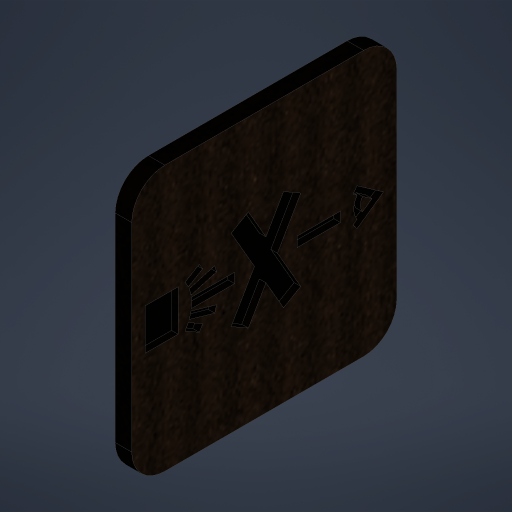
# Autodesk Inventor part: LightGateCard_V1
Saved by Autodesk Inventor 2024.1 (Build 281209000, 209)
## iProperties
Created: 2023-05-21
Part Number: LightGateCard_V1
Material: MDF Medium Density Fiberboard
Document SubType Name: Modeling
Designer: jaege
Density: 0.8 g/cm^3
Appearance: Cardboard - Corrugated
Mass: 4.78727 g
Surface Area: 45.5722 cm^2
Volume: 5.98408 cm^3
Author: jaege
## iProperties of the stored document LightGateCard_3DPrint.ipt
Created: 2023-08-10
Part Number: LightGateCard_3DPrint
Material: Generic
Document SubType Name: Modeling
Designer: jaege
Density: 1 g/cm^3
Appearance: Default
Author: jaege
Autodesk Inventor part; units mm, degrees
ref_plane "YZ Plane" through (0, 0, 0) normal (1, 0, 0) x (0, 1, 0)
ref_plane "XZ Plane" through (0, 0, 0) normal (0, 1, 0) x (-1, 0, 0)
ref_plane "XY Plane" through (0, 0, 0) normal (0, 0, 1) x (1, 0, 0)
sketch "Sketch1" plane through (0, 0, 0) normal (1, 0, 0) x (0, 1, 0)
  line L0 (-20, -20) -> (20, -20)
  line L1 (20, -20) -> (20, 20)
  line L2 (20, 20) -> (-20, 20)
  line L3 (-20, 20) -> (-20, -20)
  line L4 (-20, -20) -> (20, 20) construction
  line L5 (20, -20) -> (-20, 20) construction
  point P0 (0, 0)
  dimension "d1" = 40
  dimension "d2" = 40
  constraints: 12 end point, 2 midpoint, 2 parallel, 1 horizontal, 1 perpendicular
  measures "d1" distance of L0.start L0.end
  measures "d2" distance of L0.end L1.end
extrude "Outline" add sketch "Sketch1" along normal blind 2.5
sketch "Sketch2" plane through (2.5, 0, 0) normal (1, 0, 0) x (0, 0, -1)
  line L0 (20, 20) -> (-20, 20) projected
  line L1 (20, -20) -> (20, 20) projected
  line L2 (-18, 3.1) -> (-13, 3.1)
  line L3 (-13, 3.1) -> (-13, -3.1)
  line L4 (-13, -3.1) -> (-18, -3.1)
  line L5 (-18, -3.1) -> (-18, 3.1)
  line L6 (-11, 0.75) -> (-4.4788, 0.75)
  line L7 (-4.4788, 0.75) -> (-4.4788, -0.75)
  line L8 (-4.4788, -0.75) -> (-11, -0.75)
  line L9 (-11, -0.75) -> (-11, 0.75)
  line L10 (13.9738, 2.8192) -> (18, 0)
  line L11 (18, 0) -> (13.9738, -2.8192)
  line L12 (13.9738, 2.8192) -> (13.4003, 2)
  line L13 (13.4003, 2) -> (16.2566, 0)
  line L14 (16.2566, 0) -> (13.4003, -2)
  line L15 (13.4003, -2) -> (13.9738, -2.8192)
  line L16 (-18, 0) -> (16.2566, 0) construction
  arc A0 (14.0039, 1.5773) -> (14.0039, -1.5773) centre (16.2566, 0) ccw
  arc A1 (14.823, 1.0038) -> (14.823, -1.0038) centre (16.2566, 0) ccw
  line L17 (4.9853, 0.75) -> (11.5066, 0.75)
  line L18 (11.5066, 0.75) -> (11.5066, -0.75)
  line L19 (11.5066, -0.75) -> (4.9853, -0.75)
  line L20 (4.9853, -0.75) -> (4.9853, 0.75)
  line L21 (-11.3236, 2.0044) -> (-11.048, 1.0432)
  line L22 (-11.048, 1.0432) -> (-7.203, 2.1457)
  line L23 (-7.203, 2.1457) -> (-7.4786, 3.107)
  line L24 (-7.4786, 3.107) -> (-11.3236, 2.0044)
  line L25 (-11.048, -1.0432) -> (-7.203, -2.1457)
  line L26 (-7.203, -2.1457) -> (-7.4786, -3.107)
  line L27 (-7.4786, -3.107) -> (-11.3236, -2.0044)
  line L28 (-11.3236, -2.0044) -> (-11.048, -1.0432)
  circle A2 centre (-16.5, 0) radius 5.5509 construction
  line L29 (-11.9623, 3.1972) -> (-11.4623, 2.3312)
  line L30 (-11.4623, 2.3312) -> (-9.2973, 3.5812)
  line L31 (-9.2973, 3.5812) -> (-9.7973, 4.4472)
  line L32 (-9.7973, 4.4472) -> (-11.9623, 3.1972)
  line L33 (-11.4623, -2.3312) -> (-11.9623, -3.1972)
  line L34 (-11.9623, -3.1972) -> (-9.7973, -4.4472)
  line L35 (-9.7973, -4.4472) -> (-9.2973, -3.5812)
  line L36 (-9.2973, -3.5812) -> (-11.4623, -2.3312)
  line L37 (-4.9984, 6.0961) -> (-2.4003, 7.5961)
  line L38 (-2.4003, 7.5961) -> (5.5049, -6.0961)
  line L39 (5.5049, -6.0961) -> (2.9068, -7.5961)
  line L40 (2.9068, -7.5961) -> (-4.9984, 6.0961)
  line L41 (-4.9984, -6.0961) -> (2.9068, 7.5961)
  line L42 (2.9068, 7.5961) -> (5.5049, 6.0961)
  line L43 (5.5049, 6.0961) -> (-2.4003, -7.5961)
  line L44 (-2.4003, -7.5961) -> (-4.9984, -6.0961)
  line L45 (-4.9984, 7.5961) -> (5.5049, 7.5961) construction
  line L46 (5.5049, 7.5961) -> (5.5049, -7.5961) construction
  line L47 (5.5049, -7.5961) -> (-4.9984, -7.5961) construction
  line L48 (-4.9984, -7.5961) -> (-4.9984, 7.5961) construction
  line L49 (-20, -20) -> (20, -20) projected
  line L50 (-20, 20) -> (-20, -20) projected
  line L51 (-4.9984, 6.0961) -> (-11, 6.0961) construction
  line L52 (5.5049, 6.0961) -> (11.5066, 6.0961) construction
  point P0 (0, 0)
  point P1 (-13, 0)
  point P2 (-11, 0)
  point P3 (13.5066, 0)
  point P4 (-1.0458, 0.75)
  point P5 (1.5523, 0.75)
  point P6 (0.2533, -7.5961)
  point P7 (11.5066, 0)
  point P8 (5.5049, 0)
  point P9 (4.9853, 0)
  point P10 (-1.4788, 0)
  point P11 (0.2533, -3)
  point P12 (1.9853, 0)
  point P13 (0.2533, 3)
  point P14 (20, 0)
  dimension "d12" = 35
  dimension "d13" = 35
  dimension "d14" = 4
  dimension "d15" = 1
  dimension "d16" = 1
  dimension "d17" = 2.75
  dimension "d18" = 1.5
  dimension "d19" = 2
  dimension "d21" = 5
  dimension "d22" = 2
  dimension "d23" = 1
  dimension "d24" = 1
  dimension "d25" = 3.5
  dimension "d26" = 16
  dimension "d27" = 16
  dimension "d28" = 4
  dimension "d29" = 2.5
  dimension "d30" = 1
  dimension "d31" = 14
  dimension "d32" = 14
  dimension "d33" = 1
  dimension "d34" = 2.5
  dimension "d35" = 6.2
  dimension "d36" = 60
  dimension "d37" = 60
  dimension "d38" = 3
  dimension "d40" = 2
  dimension "d41" = 2
  dimension "d42" = 3
  dimension "d45" = 15.1922
  constraints: 98 end point, 22 parallel, 12 perpendicular, 10 midpoint, 7 horizontal, 7 horizontal alignment, 7 point on line, 6 vertical alignment, 5 equal length, 5 point on circle, 2 centre point, 2 collinear, 1 concentric, 11 other
  measures "d12" angle of L10 L16
  measures "d13" angle of L11 L16
  measures "d14" distance of L14.end L13.start
  measures "d15" radial gap between concentric circles of A1 A0
  measures "d16" distance between parallel lines of L10 L13
  measures "d17" radius of A0
  measures "d18" distance of L8.end L6.start
  measures "d19" distance from line of point (13.507, 0) L18
  measures "d21" distance between parallel lines of L5 L3
  measures "d22" distance between parallel lines of L3 L9
  measures "d23" distance of L23.start L23.end
  measures "d24" distance of L26.start L26.end
  measures "d25" distance from line of L3 point (-16.5, 0)
  measures "d26" angle of L25 L8
  measures "d27" angle of L22 L6
  measures "d28" distance of L23.end L24.end
  measures "d29" distance of L31.start L29.end
  measures "d30" distance of L31.start L31.end
  measures "d31" angle of L24 L30
  measures "d32" angle of L27 L36
  measures "d33" distance of L35.start L36.start
  measures "d34" distance of L36.start L33.start
  measures "d35" distance of L4.end L2.start
  measures "d36" angle of L38 L41
  measures "d37" angle of L6 L41
  measures "d38" distance of L37.start L37.end
  measures "d40" distance between parallel lines of L50 L5
  measures "d41" distance from line of L1 L10.end
  measures "d42" distance from line of point (-1.479, 0) L7
  measures "d45" distance of L45.end L46.end
extrude "Extrusion2" cut sketch "Sketch2" against normal blind 1 contours L2 L3 L4 L5 | L6 L7 L8 L9 | L10 L11 L15 L14 L13 L12 | L13 A1 L14 A0 | L17 L18 L19 L20 | L24 L23 L22 L21 | L25 L26 L27 L28 | L32 L31 L30 L29 | L36 L35 L34 L33 | L37 L38 L41 L40 | L41 L38 L43 L40 | L40 L43 L44 L41 | L41 L42 L43 L38 | L43 L38 L39 L40
sketch "Sketch4" plane through (1.5, 0, 0) normal (1, 0, 0) x (0, 0, -1)
  line L0 (-11.3236, 2.0044) -> (-11.048, 1.0432) projected
  line L1 (-11.048, 1.0432) -> (-7.203, 2.1457) projected
  line L2 (-7.203, 2.1457) -> (-7.4786, 3.107) projected
  line L3 (-7.4786, 3.107) -> (-11.3236, 2.0044) projected
  line L4 (0.2533, -3) -> (2.9068, -7.5961) projected
  line L5 (2.9068, -7.5961) -> (5.5049, -6.0961) projected
  line L6 (5.5049, -6.0961) -> (1.9853, 0) projected
  line L7 (1.9853, 0) -> (5.5049, 6.0961) projected
  line L8 (5.5049, 6.0961) -> (2.9068, 7.5961) projected
  line L9 (2.9068, 7.5961) -> (0.2533, 3) projected
  line L10 (0.2533, 3) -> (-2.4003, 7.5961) projected
  line L11 (-2.4003, 7.5961) -> (-4.9984, 6.0961) projected
  line L12 (-4.9984, 6.0961) -> (-1.4788, 0) projected
  line L13 (-1.4788, 0) -> (-4.9984, -6.0961) projected
  line L14 (-4.9984, -6.0961) -> (-2.4003, -7.5961) projected
  line L15 (-2.4003, -7.5961) -> (0.2533, -3) projected
  line L16 (11.5066, 0.75) -> (4.9853, 0.75) projected
  line L17 (4.9853, 0.75) -> (4.9853, -0.75) projected
  line L18 (4.9853, -0.75) -> (11.5066, -0.75) projected
  line L19 (11.5066, -0.75) -> (11.5066, 0.75) projected
  line L20 (-9.2973, 3.5812) -> (-9.7973, 4.4472) projected
  line L21 (-9.7973, 4.4472) -> (-11.9623, 3.1972) projected
  line L22 (-11.9623, 3.1972) -> (-11.4623, 2.3312) projected
  line L23 (-11.4623, 2.3312) -> (-9.2973, 3.5812) projected
  line L24 (-4.4788, -0.75) -> (-4.4788, 0.75) projected
  line L25 (-4.4788, 0.75) -> (-11, 0.75) projected
  line L26 (-11, 0.75) -> (-11, -0.75) projected
  line L27 (-11, -0.75) -> (-4.4788, -0.75) projected
  line L28 (-9.7973, -4.4472) -> (-9.2973, -3.5812) projected
  line L29 (-9.2973, -3.5812) -> (-11.4623, -2.3312) projected
  line L30 (-11.4623, -2.3312) -> (-11.9623, -3.1972) projected
  line L31 (-11.9623, -3.1972) -> (-9.7973, -4.4472) projected
  line L32 (14.823, 1.0038) -> (16.2566, 0) projected
  line L33 (16.2566, 0) -> (14.823, -1.0038) projected
  arc A0 (14.823, 1.0038) -> (14.823, -1.0038) centre (16.2566, 0) ccw projected
  line L34 (13.9738, -2.8192) -> (18, 0) projected
  line L35 (18, 0) -> (13.9738, 2.8192) projected
  line L36 (13.9738, 2.8192) -> (13.4003, 2) projected
  line L37 (13.4003, 2) -> (14.0039, 1.5773) projected
  arc A1 (14.0039, 1.5773) -> (14.0039, -1.5773) centre (16.2566, 0) ccw projected
  line L38 (14.0039, -1.5773) -> (13.4003, -2) projected
  line L39 (13.4003, -2) -> (13.9738, -2.8192) projected
  line L40 (-11.3236, -2.0044) -> (-7.4786, -3.107) projected
  line L41 (-7.4786, -3.107) -> (-7.203, -2.1457) projected
  line L42 (-7.203, -2.1457) -> (-11.048, -1.0432) projected
  line L43 (-11.048, -1.0432) -> (-11.3236, -2.0044) projected
  line L44 (-13, -3.1) -> (-13, 3.1) projected
  line L45 (-13, 3.1) -> (-18, 3.1) projected
  line L46 (-18, 3.1) -> (-18, -3.1) projected
  line L47 (-18, -3.1) -> (-13, -3.1) projected
  line L48 (20, 20) -> (20, -20) projected
  line L49 (20, -20) -> (-20, -20) projected
  line L50 (-20, -20) -> (-20, 20) projected
  line L51 (-20, 20) -> (20, 20) projected
  point P0 (0, 0)
fillet "Fillet1" radius 5 4 edges at (1.25, 20, -20) (1.25, -20, -20) (1.25, 20, 20) (1.25, -20, 20)
sketch "Sketch5" plane through (2.5, 0, 0) normal (1, 0, 0) x (0, 0, -1)
  arc A0 (-20, -15) -> (-15, -20) centre (-15, -15) ccw projected
  line L0 (-20, -15) -> (-20, 15) projected
  arc A1 (-15, 20) -> (-20, 15) centre (-15, 15) ccw projected
  line L1 (-15, 20) -> (15, 20) projected
  arc A2 (20, 15) -> (15, 20) centre (15, 15) ccw projected
  line L2 (20, 15) -> (20, -15) projected
  arc A3 (15, -20) -> (20, -15) centre (15, -15) ccw projected
  line L3 (15, -20) -> (-15, -20) projected
  line L4 (-13, -3.1) -> (-13, 3.1) projected
  line L5 (-13, 3.1) -> (-18, 3.1) projected
  line L6 (-18, 3.1) -> (-18, -3.1) projected
  line L7 (-18, -3.1) -> (-13, -3.1) projected
  line L8 (-11.3236, -2.0044) -> (-7.4786, -3.107) projected
  line L9 (-7.4786, -3.107) -> (-7.203, -2.1457) projected
  line L10 (-7.203, -2.1457) -> (-11.048, -1.0432) projected
  line L11 (-11.048, -1.0432) -> (-11.3236, -2.0044) projected
  line L12 (13.9738, -2.8192) -> (18, 0) projected
  line L13 (18, 0) -> (13.9738, 2.8192) projected
  line L14 (13.9738, 2.8192) -> (13.4003, 2) projected
  line L15 (13.4003, 2) -> (14.0039, 1.5773) projected
  arc A4 (14.0039, 1.5773) -> (14.0039, -1.5773) centre (16.2566, 0) ccw projected
  line L16 (14.0039, -1.5773) -> (13.4003, -2) projected
  line L17 (13.4003, -2) -> (13.9738, -2.8192) projected
  line L18 (-9.7973, -4.4472) -> (-9.2973, -3.5812) projected
  line L19 (-9.2973, -3.5812) -> (-11.4623, -2.3312) projected
  line L20 (-11.4623, -2.3312) -> (-11.9623, -3.1972) projected
  line L21 (-11.9623, -3.1972) -> (-9.7973, -4.4472) projected
  line L22 (-4.4788, -0.75) -> (-4.4788, 0.75) projected
  line L23 (-4.4788, 0.75) -> (-11, 0.75) projected
  line L24 (-11, 0.75) -> (-11, -0.75) projected
  line L25 (-11, -0.75) -> (-4.4788, -0.75) projected
  line L26 (-9.2973, 3.5812) -> (-9.7973, 4.4472) projected
  line L27 (-9.7973, 4.4472) -> (-11.9623, 3.1972) projected
  line L28 (-11.9623, 3.1972) -> (-11.4623, 2.3312) projected
  line L29 (-11.4623, 2.3312) -> (-9.2973, 3.5812) projected
  line L30 (11.5066, 0.75) -> (4.9853, 0.75) projected
  line L31 (4.9853, 0.75) -> (4.9853, -0.75) projected
  line L32 (4.9853, -0.75) -> (11.5066, -0.75) projected
  line L33 (11.5066, -0.75) -> (11.5066, 0.75) projected
  line L34 (0.2533, -3) -> (2.9068, -7.5961) projected
  line L35 (2.9068, -7.5961) -> (5.5049, -6.0961) projected
  line L36 (5.5049, -6.0961) -> (1.9853, 0) projected
  line L37 (1.9853, 0) -> (5.5049, 6.0961) projected
  line L38 (5.5049, 6.0961) -> (2.9068, 7.5961) projected
  line L39 (2.9068, 7.5961) -> (0.2533, 3) projected
  line L40 (0.2533, 3) -> (-2.4003, 7.5961) projected
  line L41 (-2.4003, 7.5961) -> (-4.9984, 6.0961) projected
  line L42 (-4.9984, 6.0961) -> (-1.4788, 0) projected
  line L43 (-1.4788, 0) -> (-4.9984, -6.0961) projected
  line L44 (-4.9984, -6.0961) -> (-2.4003, -7.5961) projected
  line L45 (-2.4003, -7.5961) -> (0.2533, -3) projected
  line L46 (-11.3236, 2.0044) -> (-11.048, 1.0432) projected
  line L47 (-11.048, 1.0432) -> (-7.203, 2.1457) projected
  line L48 (-7.203, 2.1457) -> (-7.4786, 3.107) projected
  line L49 (-7.4786, 3.107) -> (-11.3236, 2.0044) projected
  line L50 (14.823, 1.0038) -> (16.2566, 0) projected
  line L51 (16.2566, 0) -> (14.823, -1.0038) projected
  arc A5 (14.823, 1.0038) -> (14.823, -1.0038) centre (16.2566, 0) ccw projected
  point P0 (0, 0)
body "Solid1"
